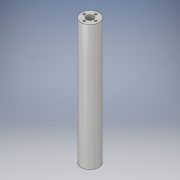
# Autodesk Inventor part: BarraSolidaMotor
Saved by Autodesk Inventor 2019 (Build 230136000, 136)
## iProperties
Created: 2019-05-15
Part Number: BarraSolidaMotor
Material: Generic
Document SubType Name: Modeling
Designer: Iván
Density: 1 g/cm^3
Appearance: Default
Author: Iván
Autodesk Inventor part; units mm, degrees
ref_plane "YZ Plane" through (0, 0, 0) normal (1, 0, 0) x (0, 1, 0)
ref_plane "XZ Plane" through (0, 0, 0) normal (0, 1, 0) x (-1, 0, 0)
ref_plane "XY Plane" through (0, 0, 0) normal (0, 0, 1) x (1, 0, 0)
sketch "Sketch1" plane through (0, 0, 0) normal (0, 1, 0) x (-1, 0, 0)
  circle A0 centre (0, 0) radius 12.7
  dimension "d0" = 25.4
  constraints: 2 coincident, 1 centre point
  measures "d0" diameter of A0
extrude "Extrusion1" add sketch "Sketch1" along normal blind 180
sketch "Sketch3" plane through (0, 180, 0) normal (0, 1, 0) x (1, 0, 0)
  point P0 (0, 0)
  point P1 (0, 0)
  constraints: 1 coincident
hole "Hole2" at (0, 180, 0) direction (0, -1, 0) diameter 10 end through all
sketch "Sketch4" plane through (0, 180, 0) normal (0, 1, 0) x (1, 0, 0)
  point P0 (0, 0)
  point P1 (0, -8.25)
  point P2 (-8.25, 0)
  point P3 (0, 8.25)
  point P4 (8.25, 0)
  dimension "d17" = 8.25
  dimension "d20" = 360
  constraints: 5 other
  measures "d17" distance of point (0, -8.25) point (0, 0)
hole "Hole3" at (0, 180, 8.25) at (-8.25, 180, 0) at (0, 180, -8.25) at (8.25, 180, 0) direction (0, -1, 0) diameter 3 depth 38.1 tip angle 118
thread "Thread1" size "M3x0.5" class "6H" standard "ANSI Metric M Profile" full length
thread "Thread2" size "M3x0.5" class "6H" standard "ANSI Metric M Profile" full length
thread "Thread3" size "M3x0.5" class "6H" standard "ANSI Metric M Profile" full length
thread "Thread4" size "M3x0.5" class "6H" standard "ANSI Metric M Profile" full length
sketch "Sketch5" plane through (0, 0, 0) normal (0, -1, 0) x (1, 0, 0)
  circle A0 centre (8.25, 0) radius 1.5 projected
  circle A1 centre (0, 8.25) radius 1.5 projected
  circle A2 centre (-8.25, 0) radius 1.5 projected
  circle A3 centre (0, -8.25) radius 1.5 projected
  point P0 (0, 0)
  constraints: 4 coincident
hole "Hole4" at (8.25, 0, 0) at (0, 0, 8.25) at (-8.25, 0, 0) at (0, 0, -8.25) direction (0, 1, 0) diameter 3 depth 25.4
thread "Thread5" size "M3x0.5" class "6H" standard "ANSI Metric M Profile" full length
thread "Thread6" size "M3x0.5" class "6H" standard "ANSI Metric M Profile" full length
thread "Thread7" size "M3x0.5" class "6H" standard "ANSI Metric M Profile" full length
thread "Thread8" size "M3x0.5" class "6H" standard "ANSI Metric M Profile" full length
body "Solid1"
